Autodesk Inventor part; units mm, degrees
note: some values were not read from the file. Chosen so that the rebuilt part matches the saved one: direction of "Hole2".
(part 18 of 20)
  ellipse E641 centre (8.105457, -1.905648) end of major axis (8.046544, -1.401076) minor radius 0.000049 (8.046544, -1.401076) -> (8.078209, -1.672645) ccw
  line L861 (7.588206, -0.94314) -> (7.98763, -0.896503)
  line L862 (8.837388, -8.177544) -> (8.078209, -1.672645)
  line L863 (8.05096, -1.439642) -> (8.81014, -7.944541)
  line L864 (8.981303, -0.780694) -> (7.987731, -0.896542)
  line L865 (8.046645, -1.401115) -> (7.987731, -0.896542)
  line L866 (8.046645, -1.401115) -> (9.040217, -1.285266)
  line L867 (9.040217, -1.285266) -> (8.981303, -0.780694)
  line L868 (8.981373, -0.780721) -> (8.981303, -0.780694)
  line L869 (7.987731, -0.896542) -> (7.98763, -0.896503)
  line L870 (8.046544, -1.401076) -> (8.046645, -1.401115)
  line L871 (-7.593552, -4.618887) -> (-7.774689, -6.528342)
  line L872 (-7.593589, -4.618889) -> (-7.662654, -5.34695)
  ellipse E642 centre (-7.593625, -4.618891) end of major axis (-7.6416, -5.124621) minor radius 0.000036 (-7.593588, -4.618887) -> (-7.57144, -4.385367) ccw
  ellipse E643 centre (-7.593625, -4.618891) end of major axis (-7.689575, -5.63035) minor radius 0.000072 (-7.593552, -4.618882) -> (-7.549255, -4.151843) ccw
  ellipse E644 centre (-6.975368, 1.901046) end of major axis (-6.879418, 2.912506) minor radius 0.000072 (-6.930999, 2.36809) -> (-6.879418, 2.912506) ccw
  ellipse E645 centre (-6.975368, 1.901046) end of major axis (-6.927393, 2.406776) minor radius 0.000036 (-6.953183, 2.134568) -> (-6.927393, 2.406776) ccw
  line L873 (-6.879418, 2.912506) -> (-4.599252, 2.696203)
  line L874 (-7.57144, -4.385369) -> (-6.953183, 2.134568)
  line L875 (-7.549256, -4.151847) -> (-6.930999, 2.36809)
  line L876 (-6.87949, 2.912501) -> (-7.875247, 3.006926)
  line L877 (-7.923221, 2.501197) -> (-7.875247, 3.006926)
  line L878 (-7.923221, 2.501197) -> (-6.927464, 2.406772)
  line L879 (-6.87949, 2.912501) -> (-6.927464, 2.406772)
  line L880 (-7.875247, 3.006926) -> (-7.875359, 3.006919)
  line L881 (-6.927464, 2.406772) -> (-6.927393, 2.406776)
  line L882 (-6.879418, 2.912506) -> (-6.87949, 2.912501)
  line L883 (-3.994803, -3.77755) -> (-3.994871, -4.67207)
  line L884 (4.005197, -3.778158) -> (4.005129, -4.672679)
  line L885 (-3.994803, -3.77755) -> (-3.994768, -3.321333)
  line L886 (4.005197, -3.778158) -> (4.005231, -3.321941)
  line L887 (4.005703, 2.876499) -> (4.005738, 3.340448)
  line L888 (-3.994262, 3.341056) -> (-3.994297, 2.877107)
  line L889 (-3.994262, 3.341056) -> (4.005738, 3.340448)
  line L890 (-3.994768, -3.321333) -> (-3.994297, 2.877107)
  line L891 (4.005703, 2.876499) -> (4.005231, -3.321941)
  line L892 (5.005708, 2.94345) -> (4.005731, 3.241593)
  line L893 (4.005692, 2.735858) -> (4.482473, 2.593706)
  line L894 (5.005692, 2.732918) -> (5.005708, 2.94345)
  line L895 (-3.994269, 3.242201) -> (-4.994292, 2.94421)
  line L896 (-4.994308, 2.733679) -> (-4.994292, 2.94421)
  line L897 (-4.47111, 2.594387) -> (-3.994308, 2.736466)
  line L898 (7.672809, -5.348116) -> (7.603854, -4.620045)
  line L899 (7.603818, -4.620042) -> (7.784664, -6.529525)
  ellipse E646 centre (7.603891, -4.620047) end of major axis (7.555992, -4.11431) minor radius 0.000036 (7.581741, -4.386522) -> (7.603854, -4.620045) ccw
  ellipse E647 centre (7.603891, -4.620047) end of major axis (7.699687, -5.631521) minor radius 0.000072 (7.559592, -4.152992) -> (7.603817, -4.620038) ccw
  ellipse E648 centre (6.986625, 1.899985) end of major axis (6.890829, 2.911458) minor radius 0.000072 (6.890829, 2.911458) -> (6.942327, 2.367035) ccw
  ellipse E649 centre (6.986625, 1.899985) end of major axis (6.938727, 2.405721) minor radius 0.000036 (6.938727, 2.405721) -> (6.964476, 2.13351) ccw
  line L900 (4.610631, 2.695502) -> (6.890829, 2.911458)
  line L901 (7.581741, -4.386522) -> (6.964476, 2.13351)
  line L902 (6.942327, 2.367035) -> (7.559592, -4.152996)
  line L903 (7.886672, 3.005727) -> (6.890901, 2.911454)
  line L904 (6.938799, 2.405717) -> (6.890901, 2.911454)
  line L905 (6.938799, 2.405717) -> (7.93457, 2.499991)
  line L906 (7.93457, 2.499991) -> (7.886672, 3.005727)
  line L907 (7.886784, 3.00572) -> (7.886672, 3.005727)
  line L908 (6.890901, 2.911454) -> (6.890829, 2.911458)
  line L909 (6.938727, 2.405721) -> (6.938799, 2.405717)
  line L910 (-7.776794, -8.27734) -> (-7.755978, -8.078526)
  line L911 (-7.75575, -8.07845) -> (-7.776577, -8.277363)
  line L912 (-7.755978, -8.078526) -> (-7.75575, -8.07845)
  line L913 (-8.025217, -8.25133) -> (-8.025445, -8.251406)
  line L914 (-7.776577, -8.277363) -> (-8.025217, -8.25133)
  line L915 (-6.782013, -8.381497) -> (-6.761187, -8.182584)
  line L916 (-6.533372, -8.40753) -> (-6.782013, -8.381497)
  line L917 (-6.731454, -10.297276) -> (-6.979877, -10.271266)
  line L918 (-6.731226, -10.2972) -> (-6.731454, -10.297276)
  line L919 (-7.000693, -10.47008) -> (-6.979867, -10.271167)
  line L920 (-6.979867, -10.271167) -> (-6.731226, -10.2972)
  line L921 (-7.000922, -10.470155) -> (-7.000693, -10.47008)
  line L922 (-7.000922, -10.470155) -> (-7.265073, -10.442498)
  line L923 (-8.208069, -9.995621) -> (-8.025445, -8.251406)
  line L924 (-7.75575, -8.07845) -> (-6.761187, -8.182584)
  line L925 (-6.533372, -8.40753) -> (-6.731226, -10.2972)
  line L926 (-8.223071, -10.141) -> (-8.025217, -8.25133)
  line L927 (-7.000693, -10.47008) -> (-7.995257, -10.365946)
  line L928 (-8.223071, -10.141) -> (-7.97443, -10.167033)
  line L929 (-7.97443, -10.167033) -> (-7.995257, -10.365946)
  line L930 (-6.80284, -8.580409) -> (-6.95904, -10.072254)
  line L931 (-6.95904, -10.072254) -> (-7.953603, -9.968121)
  line L932 (-7.953603, -9.968121) -> (-7.797403, -8.476276)
  line L933 (-7.797403, -8.476276) -> (-6.80284, -8.580409)
  line L934 (-7.11621, -9.878579) -> (-6.996733, -8.73747)
  line L935 (-6.95904, -10.072254) -> (-7.11621, -9.878579)
  line L936 (-6.80284, -8.580409) -> (-6.996733, -8.73747)
  line L937 (-6.996733, -8.73747) -> (-7.640559, -8.67006)
  line L938 (-7.797403, -8.476276) -> (-7.640559, -8.67006)
  line L939 (-7.640559, -8.67006) -> (-7.760036, -9.811168)
  line L940 (-7.953603, -9.968121) -> (-7.760036, -9.811168)
  line L941 (-7.760036, -9.811168) -> (-7.11621, -9.878579)
  circle A21 centre (-7.35107, -9.013818) radius 0.1
  line L942 (-7.517123, -9.159232) -> (-7.483402, -8.83717)
  line L943 (-7.483435, -8.837181) -> (-7.483402, -8.83717)
  line L944 (-7.517156, -9.159243) -> (-7.483435, -8.837181)
  line L945 (-7.517156, -9.159243) -> (-7.517123, -9.159232)
  line L946 (-7.483402, -8.83717) -> (-7.185033, -8.86841)
  line L947 (-7.185033, -8.86841) -> (-7.218754, -9.190472)
  line L948 (-7.218787, -9.190483) -> (-7.218754, -9.190472)
  line L949 (-7.218754, -9.190472) -> (-7.517123, -9.159232)
  line L950 (-7.218787, -9.190483) -> (-7.517156, -9.159243)
  line L951 (-6.390906, -18.904533) -> (-6.589819, -18.883707)
  line L952 (-6.390678, -18.904457) -> (-6.390906, -18.904533)
  line L953 (-6.589591, -18.883631) -> (-6.390678, -18.904457)
  line L954 (-6.589819, -18.883707) -> (-6.589591, -18.883631)
  line L955 (-6.416939, -19.153174) -> (-6.390906, -18.904533)
  line L956 (-6.416711, -19.153098) -> (-6.416939, -19.153174)
  line L957 (-6.390678, -18.904457) -> (-6.416711, -19.153098)
  line L958 (-6.286762, -17.909871) -> (-6.260739, -17.661329)
  line L959 (-6.485457, -17.889067) -> (-6.485685, -17.889143)
  line L960 (-6.286544, -17.909894) -> (-6.485457, -17.889067)
  line L961 (-6.260511, -17.661253) -> (-6.286544, -17.909894)
  line L962 (-6.260739, -17.661329) -> (-6.260511, -17.661253)
  line L963 (-6.589819, -18.883707) -> (-6.485685, -17.889143)
  line L964 (-4.527269, -19.351028) -> (-6.416939, -19.153174)
  line L965 (-6.589591, -18.883631) -> (-6.485457, -17.889067)
  line L966 (-6.260511, -17.661253) -> (-4.370841, -17.859107)
  line L967 (-4.527041, -19.350952) -> (-6.416711, -19.153098)
  line L968 (-4.197961, -18.128574) -> (-4.302095, -19.123138)
  line L969 (-4.302323, -19.123214) -> (-4.501018, -19.10241)
  line L970 (-4.527041, -19.350952) -> (-4.501008, -19.102311)
  line L971 (-4.501008, -19.102311) -> (-4.302095, -19.123138)
  line L972 (-4.302095, -19.123138) -> (-4.302323, -19.123214)
  line L973 (-4.527269, -19.351028) -> (-4.527041, -19.350952)
  line L974 (-4.197961, -18.128574) -> (-4.396874, -18.107748)
  line L975 (-4.396874, -18.107748) -> (-4.370841, -17.859107)
  line L976 (-6.087632, -17.930721) -> (-4.595787, -18.086921)
  line L977 (-4.595787, -18.086921) -> (-4.69992, -19.081484)
  line L978 (-4.69992, -19.081484) -> (-6.191765, -18.925284)
  line L979 (-6.191765, -18.925284) -> (-6.087632, -17.930721)
  line L980 (-4.78968, -18.243982) -> (-5.930788, -18.124505)
  line L981 (-4.595787, -18.086921) -> (-4.78968, -18.243982)
  line L982 (-6.087632, -17.930721) -> (-5.930788, -18.124505)
  line L983 (-5.930788, -18.124505) -> (-5.998198, -18.768332)
  line L984 (-6.191765, -18.925284) -> (-5.998198, -18.768332)
  line L985 (-5.998198, -18.768332) -> (-4.85709, -18.887809)
  line L986 (-4.69992, -19.081484) -> (-4.85709, -18.887809)
  line L987 (-4.85709, -18.887809) -> (-4.78968, -18.243982)
  circle A22 centre (-5.654386, -18.47887) radius 0.1
  line L988 (-5.508983, -18.644917) -> (-5.831045, -18.611196)
  line L989 (-5.831077, -18.611207) -> (-5.831045, -18.611196)
  line L990 (-5.509015, -18.644928) -> (-5.831077, -18.611207)
  line L991 (-5.509015, -18.644928) -> (-5.508983, -18.644917)
  line L992 (-5.831045, -18.611196) -> (-5.799805, -18.312827)
  line L993 (-5.799837, -18.312838) -> (-5.799805, -18.312827)
  line L994 (-5.831077, -18.611207) -> (-5.799837, -18.312838)
  line L995 (-5.799805, -18.312827) -> (-5.477743, -18.346548)
  line L996 (-5.477743, -18.346548) -> (-5.508983, -18.644917)
  line L997 (-3.430044, -6.945819) -> (-3.430059, -7.144732)
  line L998 (-3.430059, -7.144732) -> (-3.680059, -7.144713)
  line L999 (-2.430059, -7.144809) -> (-2.430044, -6.945895)
  line L1000 (-2.180059, -7.144828) -> (-2.430059, -7.144809)
  line L1001 (-3.430044, -6.945819) -> (-2.430044, -6.945895)
  line L1002 (-2.180059, -7.144828) -> (-2.180193, -8.902773)
  line L1003 (-3.680193, -8.902659) -> (-3.680059, -7.144713)
  line L1004 (-2.430074, -7.343723) -> (-2.430178, -8.704102)
  line L1005 (-3.430178, -8.704026) -> (-3.430074, -7.343646)
  line L1006 (-3.430074, -7.343646) -> (-2.430074, -7.343723)
  line L1007 (-2.430074, -7.343723) -> (-2.590055, -7.597215)
  line L1008 (-3.430074, -7.343646) -> (-3.270133, -7.597163)
  ellipse E650 centre (-2.930117, -7.907177) end of major axis (-2.830117, -7.907184) minor radius 0.099457
  ellipse E651 centre (-2.930118, -7.91238) end of major axis (-2.830118, -7.912388) minor radius 0.099457 (-3.030118, -7.912373) -> (-2.830118, -7.912388) ccw
  line L1009 (-3.030118, -7.912373) -> (-3.030117, -7.907169)
  line L1010 (-2.830118, -7.912388) -> (-2.830117, -7.907184)
  line L1011 (-3.08013, -8.073401) -> (-3.080105, -7.751337)
  line L1012 (-3.080131, -8.083948) -> (-3.08013, -8.073401)
  line L1013 (-3.080105, -7.751337) -> (-2.780105, -7.751359)
  line L1014 (-2.780105, -7.751359) -> (-2.78013, -8.073424)
  line L1015 (-2.780131, -8.083971) -> (-2.78013, -8.073424)
  line L1016 (-2.78013, -8.073424) -> (-3.08013, -8.073401)
  line L1017 (-1.145848, -17.513296) -> (-0.945848, -17.513311)
  line L1018 (-1.145854, -17.595223) -> (-1.145848, -17.513296)
  line L1019 (-0.945867, -17.761954) -> (-0.945873, -17.843571)
  line L1020 (-0.945848, -17.513311) -> (-0.945867, -17.761954)
  line L1021 (-0.945772, -16.518742) -> (-1.145772, -16.518726)
  line L1022 (-0.945753, -16.270099) -> (-0.945772, -16.518742)
  line L1023 (-1.145848, -17.513296) -> (-1.145772, -16.518726)
  line L1024 (-0.945753, -16.270099) -> (0.954247, -16.270244)
  line L1025 (0.954133, -17.762098) -> (-0.945867, -17.761954)
  line L1026 (1.154228, -16.518901) -> (1.154152, -17.513471)
  line L1027 (0.954133, -17.762098) -> (0.954152, -17.513456)
  line L1028 (0.954152, -17.513456) -> (1.154152, -17.513471)
  line L1029 (1.154152, -17.513471) -> (1.154146, -17.595398)
  line L1030 (0.954127, -17.843715) -> (0.954133, -17.762098)
  line L1031 (1.154228, -16.518901) -> (0.954228, -16.518886)
  line L1032 (0.954228, -16.518886) -> (0.954247, -16.270244)
  line L1033 (-0.745772, -16.518757) -> (0.754228, -16.518871)
  line L1034 (0.754228, -16.518871) -> (0.754152, -17.513441)
  line L1035 (0.754152, -17.513441) -> (-0.745848, -17.513327)
  line L1036 (-0.745848, -17.513327) -> (-0.745772, -16.518757)
  line L1037 (0.754228, -16.518871) -> (0.613598, -16.741703)
  line L1038 (-0.745772, -16.518757) -> (-0.605176, -16.74161)
  line L1039 (-0.745848, -17.513327) -> (-0.606744, -17.457092)
  line L1040 (0.754152, -17.513441) -> (0.615057, -17.457185)
  ellipse E652 centre (-0.257727, -17.094133) end of major axis (-0.157727, -17.09414) minor radius 0.099457
  line L1041 (-0.357728, -17.098618) -> (-0.357727, -17.094125)
  line L1042 (-0.157728, -17.098634) -> (-0.157727, -17.09414)
  line L1043 (4.509081, -19.103095) -> (4.310383, -19.123869)
  line L1044 (4.310154, -19.123793) -> (4.50907, -19.102996)
  line L1045 (4.310383, -19.123869) -> (4.310154, -19.123793)
  line L1046 (4.535066, -19.351641) -> (4.535294, -19.351717)
  line L1047 (4.50907, -19.102996) -> (4.535066, -19.351641)
  line L1048 (4.405088, -18.108417) -> (4.206172, -18.129214)
  line L1049 (4.379093, -17.859772) -> (4.405088, -18.108417)
  line L1050 (6.269021, -17.662282) -> (6.295006, -17.910828)
  line L1051 (6.268793, -17.662206) -> (6.269021, -17.662282)
  line L1052 (6.493704, -17.890055) -> (6.294789, -17.910851)
  line L1053 (6.294789, -17.910851) -> (6.268793, -17.662206)
  line L1054 (6.493932, -17.89013) -> (6.493704, -17.890055)
  line L1055 (6.493932, -17.89013) -> (6.597915, -18.88471)
  line L1056 (6.424994, -19.154151) -> (4.535294, -19.351717)
  line L1057 (4.310154, -19.123793) -> (4.206172, -18.129214)
  line L1058 (4.379093, -17.859772) -> (6.268793, -17.662206)
  line L1059 (6.424766, -19.154075) -> (4.535066, -19.351641)
  line L1060 (6.493704, -17.890055) -> (6.597687, -18.884634)
  line L1061 (6.597915, -18.88471) -> (6.398999, -18.905506)
  line L1062 (6.398999, -18.905506) -> (6.424994, -19.154151)
  line L1063 (6.424766, -19.154075) -> (6.398771, -18.90543)
  line L1064 (6.398771, -18.90543) -> (6.597687, -18.884634)
  line L1065 (6.597687, -18.884634) -> (6.597915, -18.88471)
  line L1066 (6.398771, -18.90543) -> (6.398999, -18.905506)
  line L1067 (6.424994, -19.154151) -> (6.424766, -19.154075)
  line L1068 (4.604004, -18.087621) -> (6.095873, -17.931647)
  line L1069 (6.095873, -17.931647) -> (6.199855, -18.926227)
  line L1070 (6.199855, -18.926227) -> (4.707986, -19.0822)
  line L1071 (4.707986, -19.0822) -> (4.604004, -18.087621)
  line L1072 (5.938999, -18.125408) -> (4.797873, -18.244711)
  line L1073 (6.095873, -17.931647) -> (5.938999, -18.125408)
  line L1074 (4.604004, -18.087621) -> (4.797873, -18.244711)
  line L1075 (4.797873, -18.244711) -> (4.865185, -18.888548)
  line L1076 (4.707986, -19.0822) -> (4.865185, -18.888548)
  line L1077 (4.865185, -18.888548) -> (6.006312, -18.769245)
  line L1078 (6.199855, -18.926227) -> (6.006312, -18.769245)
  line L1079 (6.006312, -18.769245) -> (5.938999, -18.125408)
  circle A23 centre (5.14156, -18.534198) radius 0.1
  line L1080 (5.318199, -18.666552) -> (4.996132, -18.700224)
  line L1081 (4.996164, -18.700235) -> (4.996132, -18.700224)
  line L1082 (5.318232, -18.666563) -> (4.996164, -18.700235)
  line L1083 (5.318232, -18.666563) -> (5.318199, -18.666552)
  line L1084 (4.996132, -18.700224) -> (4.964937, -18.40185)
  line L1085 (4.964937, -18.40185) -> (5.287004, -18.368178)
  line L1086 (5.287037, -18.368189) -> (5.287004, -18.368178)
  line L1087 (5.287004, -18.368178) -> (5.318199, -18.666552)
  line L1088 (5.287037, -18.368189) -> (5.318232, -18.666563)
  line L1089 (-1.146141, -21.369416) -> (-0.946141, -21.369432)
  line L1090 (-0.946141, -21.369432) -> (-0.94616, -21.619432)
  line L1091 (-0.946065, -20.369432) -> (-1.146065, -20.369416)
  line L1092 (-0.946054, -20.223706) -> (-0.946065, -20.369432)
  line L1093 (-1.146141, -21.369416) -> (-1.146065, -20.369416)
  line L1094 (0.95384, -21.619576) -> (-0.94616, -21.619432)
  line L1095 (1.153935, -20.369591) -> (1.153859, -21.369591)
  line L1096 (0.95384, -21.619576) -> (0.953859, -21.369576)
  line L1097 (0.953859, -21.369576) -> (1.153859, -21.369591)
  line L1098 (1.153935, -20.369591) -> (0.953935, -20.369576)
  line L1099 (0.953935, -20.369576) -> (0.953946, -20.22385)
  line L1100 (-0.746065, -20.369447) -> (0.753935, -20.369561)
  line L1101 (0.753935, -20.369561) -> (0.753859, -21.369561)
  line L1102 (0.753859, -21.369561) -> (-0.746141, -21.369447)
  line L1103 (-0.746141, -21.369447) -> (-0.746065, -20.369447)
  line L1104 (0.577595, -20.545874) -> (-0.569751, -20.545787)
  line L1105 (0.753935, -20.369561) -> (0.577595, -20.545874)
  line L1106 (-0.746065, -20.369447) -> (-0.569751, -20.545787)
  line L1107 (-0.569751, -20.545787) -> (-0.569801, -21.193133)
  line L1108 (-0.746141, -21.369447) -> (-0.569801, -21.193133)
  line L1109 (-0.569801, -21.193133) -> (0.577545, -21.193221)
  line L1110 (0.753859, -21.369561) -> (0.577545, -21.193221)
  line L1111 (0.577545, -21.193221) -> (0.577595, -20.545874)
  circle A24 centre (-0.258014, -20.869484) radius 0.1
  line L1112 (-0.096114, -21.019496) -> (-0.419937, -21.019472)
  line L1113 (-0.419937, -21.019472) -> (-0.419914, -20.719472)
  line L1114 (-0.419914, -20.719472) -> (-0.096092, -20.719496)
  line L1115 (-0.096092, -20.719496) -> (-0.096114, -21.019496)
  line L1116 (-1.146233, -22.580088) -> (-0.946233, -22.580104)
  line L1117 (-0.946233, -22.580104) -> (-0.946252, -22.828417)
  line L1118 (-1.146233, -22.580088) -> (-1.146198, -22.119416)
  line L1119 (0.953748, -22.828561) -> (-0.946252, -22.828417)
  line L1120 (1.153802, -22.119591) -> (1.153767, -22.580263)
  line L1121 (0.953748, -22.828561) -> (0.953767, -22.580248)
  line L1122 (0.953767, -22.580248) -> (1.153767, -22.580263)
  line L1123 (0.753802, -22.119561) -> (0.753767, -22.580233)
  line L1124 (0.753767, -22.580233) -> (-0.746233, -22.580119)
  line L1125 (-0.746233, -22.580119) -> (-0.746198, -22.119447)
  line L1126 (-0.569871, -22.11946) -> (-0.569884, -22.289016)
  line L1127 (-0.746233, -22.580119) -> (-0.569884, -22.289016)
  line L1128 (-0.569884, -22.289016) -> (0.577462, -22.289103)
  line L1129 (0.753767, -22.580233) -> (0.577462, -22.289103)
  line L1130 (0.577462, -22.289103) -> (0.577475, -22.119548)
  line L1131 (-0.0962, -22.139747) -> (-0.420022, -22.139722)
  line L1132 (-0.420022, -22.139722) -> (-0.420021, -22.119472)
  line L1133 (-0.096198, -22.119496) -> (-0.0962, -22.139747)
  line L1134 (-8.467791, -9.965256) -> (-8.491015, -10.163903)
  line L1135 (-8.467932, -9.96531) -> (-8.467791, -9.965256)
  line L1136 (-8.739324, -10.134872) -> (-8.739466, -10.134927)
  line L1137 (-8.491015, -10.163903) -> (-8.739324, -10.134872)
  line L1138 (-8.707345, -12.252986) -> (-8.735015, -12.249751)
  line L1139 (-8.960099, -12.022073) -> (-8.739466, -10.134927)
  line L1140 (-8.467791, -9.965256) -> (-8.207852, -9.995646)
  line L1141 (-7.265061, -10.4424) -> (-7.470105, -12.196203)
  line L1142 (-8.959957, -12.022019) -> (-8.739324, -10.134872)
  line L1143 (-7.741638, -12.365819) -> (-8.734873, -12.249696)
  line L1144 (-8.735015, -12.249751) -> (-8.723713, -12.15308)
  line L1145 (-8.739665, -12.047845) -> (-8.960099, -12.022073)
  line L1146 (-8.959957, -12.022019) -> (-8.711649, -12.051049)
  line L1147 (-8.711649, -12.051049) -> (-8.734873, -12.249696)
  line L1148 (-8.734873, -12.249696) -> (-8.735015, -12.249751)
  line L1149 (-8.711649, -12.051049) -> (-8.71179, -12.051104)
  line L1150 (-8.960099, -12.022073) -> (-8.959957, -12.022019)
  line L1151 (-7.470105, -12.196203) -> (-7.470246, -12.196257)
  line L1152 (-7.741638, -12.365819) -> (-7.718414, -12.167172)
  line L1153 (-7.718414, -12.167172) -> (-7.470105, -12.196203)
  line L1154 (-7.74178, -12.365873) -> (-7.741638, -12.365819)
  line L1155 (-7.521005, -10.478673) -> (-7.695189, -11.968525)
  line L1156 (-7.695189, -11.968525) -> (-8.688424, -11.852402)
  line L1157 (-8.688424, -11.852402) -> (-8.51424, -10.36255)
  line L1158 (-8.51424, -10.36255) -> (-7.521005, -10.478673)
  line L1159 (-7.849949, -11.772954) -> (-7.716716, -10.63337)
  line L1160 (-7.695189, -11.968525) -> (-7.849949, -11.772954)
  line L1161 (-7.521005, -10.478673) -> (-7.716716, -10.63337)
  line L1162 (-7.716716, -10.63337) -> (-8.359683, -10.558199)
  line L1163 (-8.51424, -10.36255) -> (-8.359683, -10.558199)
  line L1164 (-8.359683, -10.558199) -> (-8.492916, -11.697783)
  line L1165 (-8.688424, -11.852402) -> (-8.492916, -11.697783)
  line L1166 (-8.492916, -11.697783) -> (-7.849949, -11.772954)
  circle A25 centre (-8.074377, -10.905427) radius 0.1
  line L1167 (-8.242168, -11.048827) -> (-8.204565, -10.727195)
  line L1168 (-8.204585, -10.727202) -> (-8.204565, -10.727195)
  line L1169 (-8.242189, -11.048835) -> (-8.204585, -10.727202)
  line L1170 (-8.242189, -11.048835) -> (-8.242168, -11.048827)
  line L1171 (-8.204565, -10.727195) -> (-7.906595, -10.762032)
  line L1172 (-7.906595, -10.762032) -> (-7.944198, -11.083664)
  line L1173 (-7.944218, -11.083671) -> (-7.944198, -11.083664)
  line L1174 (-7.944198, -11.083664) -> (-8.242168, -11.048827)
  line L1175 (-7.944218, -11.083671) -> (-8.242189, -11.048835)
  line L1176 (-7.233548, -20.806996) -> (-7.432195, -20.783772)
  line L1177 (-7.233407, -20.806942) -> (-7.233548, -20.806996)
  line L1178 (-7.432054, -20.783717) -> (-7.233407, -20.806942)
  line L1179 (-7.432195, -20.783772) -> (-7.432054, -20.783717)
  line L1180 (-7.262579, -21.055305) -> (-7.233548, -20.806996)
  line L1181 (-7.262437, -21.05525) -> (-7.262579, -21.055305)
  line L1182 (-7.233407, -20.806942) -> (-7.262437, -21.05525)
  line L1183 (-7.117417, -19.813691) -> (-7.090722, -19.585361)
  line L1184 (-7.315931, -19.790482) -> (-7.316072, -19.790537)
  line L1185 (-7.117284, -19.813707) -> (-7.315931, -19.790482)
  line L1186 (-7.088253, -19.565398) -> (-7.117284, -19.813707)
  line L1187 (-7.088395, -19.565452) -> (-7.088253, -19.565398)
  line L1188 (-7.432195, -20.783772) -> (-7.316072, -19.790537)
  line L1189 (-5.375433, -21.275938) -> (-7.262579, -21.055305)
  line L1190 (-7.432054, -20.783717) -> (-7.315931, -19.790482)
  line L1191 (-7.088253, -19.565398) -> (-5.201107, -19.786031)
  line L1192 (-5.375291, -21.275884) -> (-7.262437, -21.05525)
  line L1193 (-5.031491, -20.057565) -> (-5.147613, -21.050799)
  line L1194 (-5.147755, -21.050854) -> (-5.346269, -21.027645)
  line L1195 (-5.375291, -21.275884) -> (-5.34626, -21.027575)
  line L1196 (-5.34626, -21.027575) -> (-5.147613, -21.050799)
  line L1197 (-5.147613, -21.050799) -> (-5.147755, -21.050854)
  line L1198 (-5.375433, -21.275938) -> (-5.375291, -21.275884)
  line L1199 (-5.031491, -20.057565) -> (-5.230138, -20.03434)
  line L1200 (-5.230138, -20.03434) -> (-5.201107, -19.786031)
  line L1201 (-6.918637, -19.836931) -> (-5.428785, -20.011115)
  line L1202 (-5.428785, -20.011115) -> (-5.544907, -21.00435)
  line L1203 (-5.544907, -21.00435) -> (-7.03476, -20.830166)
  line L1204 (-7.03476, -20.830166) -> (-6.918637, -19.836931)
  line L1205 (-5.624495, -20.165813) -> (-6.76408, -20.03258)
  line L1206 (-5.428785, -20.011115) -> (-5.624495, -20.165813)
  line L1207 (-6.918637, -19.836931) -> (-6.76408, -20.03258)
  line L1208 (-6.76408, -20.03258) -> (-6.839251, -20.675547)
  line L1209 (-7.03476, -20.830166) -> (-6.839251, -20.675547)
  line L1210 (-6.839251, -20.675547) -> (-5.699667, -20.80878)
  line L1211 (-5.544907, -21.00435) -> (-5.699667, -20.80878)
  line L1212 (-5.699667, -20.80878) -> (-5.624495, -20.165813)
  circle A26 centre (-6.491988, -20.390256) radius 0.1
  line L1213 (-6.348595, -20.558045) -> (-6.670227, -20.520442)
  line L1214 (-6.670247, -20.520449) -> (-6.670227, -20.520442)
  line L1215 (-6.348615, -20.558053) -> (-6.670247, -20.520449)
  line L1216 (-6.348615, -20.558053) -> (-6.348595, -20.558045)
  line L1217 (-6.670227, -20.520442) -> (-6.63539, -20.222471)
  line L1218 (-6.63541, -20.222479) -> (-6.63539, -20.222471)
  line L1219 (-6.670247, -20.520449) -> (-6.63541, -20.222479)
  line L1220 (-6.63539, -20.222471) -> (-6.313758, -20.260074)
  line L1221 (-6.313758, -20.260074) -> (-6.348595, -20.558045)
  line L1222 (-3.430178, -8.704026) -> (-3.430193, -8.902678)
  line L1223 (-3.430193, -8.902678) -> (-3.680193, -8.902659)
  line L1224 (-2.430193, -8.902754) -> (-2.430178, -8.704102)
  line L1225 (-2.180193, -8.902773) -> (-2.430193, -8.902754)
  line L1226 (-2.180349, -10.95225) -> (-2.430349, -10.952231)
  line L1227 (-2.180336, -10.789965) -> (-2.180349, -10.95225)
  line L1228 (-2.430352, -10.988597) -> (-2.430336, -10.789946)
  line L1229 (-2.430336, -10.789946) -> (-2.180336, -10.789965)
  line L1230 (-2.430364, -11.150883) -> (-2.430352, -10.988597)
  line L1231 (-2.430364, -11.150883) -> (-3.430364, -11.150807)
  line L1232 (-3.430178, -8.704026) -> (-2.430178, -8.704102)
  line L1233 (-2.180193, -8.902773) -> (-2.180336, -10.789965)
  line L1234 (-3.680336, -10.789851) -> (-3.680193, -8.902659)
  line L1235 (-2.430352, -10.988597) -> (-3.430352, -10.988521)
  line L1236 (-3.430349, -10.952155) -> (-3.680349, -10.952136)
  line L1237 (-3.680336, -10.789851) -> (-3.430336, -10.78987)
  line L1238 (-3.430336, -10.78987) -> (-3.430352, -10.988521)
  line L1239 (-3.430352, -10.988521) -> (-3.430364, -11.150807)
  line L1240 (-3.680349, -10.952136) -> (-3.680336, -10.789851)
  line L1241 (-2.430208, -9.101406) -> (-2.430321, -10.591294)
  line L1242 (-2.430321, -10.591294) -> (-3.430321, -10.591218)
  line L1243 (-3.430321, -10.591218) -> (-3.430208, -9.10133)
  line L1244 (-3.430208, -9.10133) -> (-2.430208, -9.101406)
  line L1245 (-2.606644, -10.53206) -> (-2.606557, -9.392449)
  line L1246 (-2.430321, -10.591294) -> (-2.606644, -10.53206)
  line L1247 (-2.430208, -9.101406) -> (-2.606557, -9.392449)
  line L1248 (-2.606557, -9.392449) -> (-3.253903, -9.3924)
  line L1249 (-3.430208, -9.10133) -> (-3.253903, -9.3924)
  line L1250 (-3.253903, -9.3924) -> (-3.25399, -10.532011)
  line L1251 (-3.430321, -10.591218) -> (-3.25399, -10.532011)
  line L1252 (-3.25399, -10.532011) -> (-2.606644, -10.53206)
  ellipse E653 centre (-2.930252, -9.673105) end of major axis (-2.830252, -9.673112) minor radius 0.099326
  ellipse E654 centre (-2.930252, -9.678901) end of major axis (-2.830252, -9.678908) minor radius 0.099326 (-3.030252, -9.678893) -> (-2.830252, -9.678908) ccw
  line L1253 (-3.030252, -9.678893) -> (-3.030252, -9.673097)
  line L1254 (-2.830252, -9.678908) -> (-2.830252, -9.673112)
  line L1255 (-3.080264, -9.839709) -> (-3.08024, -9.518069)
  line L1256 (-3.080266, -9.862893) -> (-3.080264, -9.839709)
  line L1257 (-3.08024, -9.518069) -> (-2.78024, -9.518092)
  line L1258 (-2.78024, -9.518092) -> (-2.780264, -9.839732)
  line L1259 (-2.780266, -9.862916) -> (-2.780264, -9.839732)
  line L1260 (-2.780264, -9.839732) -> (-3.080264, -9.839709)
  line L1261 (-2.780266, -9.862916) -> (-3.080266, -9.862893)
  line L1262 (-0.945993, -19.419875) -> (-1.145993, -19.41986)
  line L1263 (-1.14598, -19.257574) -> (-0.94598, -19.257589)
  line L1264 (-1.145993, -19.41986) -> (-1.14598, -19.257574)
  line L1265 (-0.945999, -19.505904) -> (-0.946012, -19.66819)
  line L1266 (-0.94598, -19.257589) -> (-0.945999, -19.505904)
  line L1267 (-0.945905, -18.264331) -> (-1.145905, -18.264315)
  line L1268 (-0.945886, -18.016016) -> (-0.945905, -18.264331)
  line L1269 (1.154007, -19.420035) -> (0.954007, -19.420019)
  line L1270 (0.954001, -19.506049) -> (0.95402, -19.257734)
  line L1271 (0.95402, -19.257734) -> (1.15402, -19.257749)
  line L1272 (1.15402, -19.257749) -> (1.154007, -19.420035)
  line L1273 (0.953988, -19.668334) -> (0.954001, -19.506049)
  line L1274 (0.953988, -19.668334) -> (-0.946012, -19.66819)
  line L1275 (-1.14598, -19.257574) -> (-1.145905, -18.264315)
  line L1276 (-0.945886, -18.016016) -> (0.954114, -18.016161)
  line L1277 (0.954001, -19.506049) -> (-0.945999, -19.505904)
  line L1278 (1.154095, -18.26449) -> (1.15402, -19.257749)
  line L1279 (1.154095, -18.26449) -> (0.954095, -18.264475)
  line L1280 (0.954095, -18.264475) -> (0.954114, -18.016161)
  line L1281 (-0.745905, -18.264346) -> (0.754095, -18.26446)
  line L1282 (0.754095, -18.26446) -> (0.75402, -19.257719)
  line L1283 (0.75402, -19.257719) -> (-0.74598, -19.257605)
  line L1284 (-0.74598, -19.257605) -> (-0.745905, -18.264346)
  line L1285 (0.577746, -18.555503) -> (-0.5696, -18.555416)
  line L1286 (0.754095, -18.26446) -> (0.577746, -18.555503)
  line L1287 (-0.745905, -18.264346) -> (-0.5696, -18.555416)
  line L1288 (-0.5696, -18.555416) -> (-0.569649, -19.198398)
  line L1289 (-0.74598, -19.257605) -> (-0.569649, -19.198398)
  line L1290 (-0.569649, -19.198398) -> (0.577697, -19.198485)
  line L1291 (0.75402, -19.257719) -> (0.577697, -19.198485)
  line L1292 (0.577697, -19.198485) -> (0.577746, -18.555503)
  ellipse E655 centre (-0.257861, -18.847951) end of major axis (-0.157861, -18.847959) minor radius 0.099326
  ellipse E656 centre (-0.257861, -18.853747) end of major axis (-0.157861, -18.853755) minor radius 0.099326 (-0.357861, -18.853739) -> (-0.157861, -18.853755) ccw
  line L1293 (-0.357861, -18.853739) -> (-0.357861, -18.847943)
  line L1294 (-0.157861, -18.853755) -> (-0.157861, -18.847959)
  line L1295 (-0.095961, -19.002748) -> (-0.419784, -19.002723)
  line L1296 (-0.419786, -19.025907) -> (-0.419784, -19.002723)
  line L1297 (-0.095963, -19.025932) -> (-0.419786, -19.025907)
  line L1298 (-0.095963, -19.025932) -> (-0.095961, -19.002748)
  line L1299 (-0.419784, -19.002723) -> (-0.419761, -18.704746)
  line L1300 (-0.419761, -18.704746) -> (-0.095938, -18.70477)
  line L1301 (-0.095938, -18.70477) -> (-0.095961, -19.002748)
  line L1302 (5.354039, -21.028459) -> (5.155521, -21.051637)
  line L1303 (5.15538, -21.051583) -> (5.35403, -21.028389)
  line L1304 (5.155521, -21.051637) -> (5.15538, -21.051583)
  line L1305 (5.383023, -21.276702) -> (5.383165, -21.276756)
  line L1306 (5.35403, -21.028389) -> (5.383023, -21.276702)
  line L1307 (5.238059, -20.035136) -> (5.039408, -20.05833)
  line L1308 (5.209066, -19.786823) -> (5.238059, -20.035136)
  line L1309 (7.098712, -19.58644) -> (7.125372, -19.814774)
  line L1310 (7.096246, -19.566477) -> (7.096387, -19.566531)
  line L1311 (7.323889, -19.791595) -> (7.125238, -19.81479)
  line L1312 (7.125238, -19.81479) -> (7.096246, -19.566477)
  line L1313 (7.32403, -19.79165) -> (7.323889, -19.791595)
  line L1314 (7.32403, -19.79165) -> (7.440002, -20.784903)
  line L1315 (7.270345, -21.05641) -> (5.383165, -21.276756)
  line L1316 (5.15538, -21.051583) -> (5.039408, -20.05833)
  line L1317 (5.209066, -19.786823) -> (7.096246, -19.566477)
  line L1318 (7.270203, -21.056355) -> (5.383023, -21.276702)
  line L1319 (7.323889, -19.791595) -> (7.439861, -20.784848)
  line L1320 (7.440002, -20.784903) -> (7.241352, -20.808097)
  line L1321 (7.241352, -20.808097) -> (7.270345, -21.05641)
  line L1322 (7.270203, -21.056355) -> (7.24121, -20.808042)
  line L1323 (7.24121, -20.808042) -> (7.439861, -20.784848)
  line L1324 (7.439861, -20.784848) -> (7.440002, -20.784903)
  line L1325 (7.24121, -20.808042) -> (7.241352, -20.808097)
  line L1326 (7.270345, -21.05641) -> (7.270203, -21.056355)
  line L1327 (5.436709, -20.011942) -> (6.926588, -19.837984)
  line L1328 (6.926588, -19.837984) -> (7.04256, -20.831237)
  line L1329 (7.04256, -20.831237) -> (5.552681, -21.005194)
  line L1330 (5.552681, -21.005194) -> (5.436709, -20.011942)
  line L1331 (6.772001, -20.033609) -> (5.632396, -20.166669)
  line L1332 (6.926588, -19.837984) -> (6.772001, -20.033609)
  line L1333 (5.436709, -20.011942) -> (5.632396, -20.166669)
  line L1334 (5.632396, -20.166669) -> (5.70747, -20.809647)
  line L1335 (5.552681, -21.005194) -> (5.70747, -20.809647)
  line L1336 (5.70747, -20.809647) -> (6.847075, -20.676587)
  line L1337 (7.04256, -20.831237) -> (6.847075, -20.676587)
  line L1338 (6.847075, -20.676587) -> (6.772001, -20.033609)
  circle A27 centre (5.979566, -20.451993) radius 0.1
  line L1339 (6.157786, -20.582205) -> (5.836148, -20.61976)
  line L1340 (5.836168, -20.619767) -> (5.836148, -20.61976)
  line L1341 (6.157806, -20.582213) -> (5.836168, -20.619767)
  line L1342 (6.157806, -20.582213) -> (6.157786, -20.582205)
  line L1343 (5.836148, -20.61976) -> (5.801357, -20.321784)
  line L1344 (5.801357, -20.321784) -> (6.122994, -20.28423)
  line L1345 (6.123015, -20.284237) -> (6.122994, -20.28423)
  line L1346 (6.122994, -20.28423) -> (6.157786, -20.582205)
  line L1347 (6.123015, -20.284237) -> (6.157806, -20.582213)
  line L1348 (-7.191687, -6.365321) -> (-7.172801, -6.166231)
  line L1349 (-7.172701, -6.166225) -> (-7.191589, -6.365331)
  line L1350 (-7.172801, -6.166231) -> (-7.172701, -6.166225)
  line L1351 (-7.440471, -6.341721) -> (-7.440572, -6.341727)
  line L1352 (-7.191589, -6.365331) -> (-7.440471, -6.341721)
  line L1353 (-6.196058, -6.45977) -> (-6.17717, -6.260664)
  line L1354 (-5.947175, -6.483379) -> (-6.196058, -6.45977)
  line L1355 (-7.461453, -6.561848) -> (-7.440572, -6.341727)
  line L1356 (-7.172701, -6.166225) -> (-6.17717, -6.260664)
  line L1357 (-5.947175, -6.483379) -> (-6.126609, -8.374888)
  line L1358 (-7.606703, -8.094056) -> (-7.440471, -6.341721)
  line L1359 (-6.39438, -8.550384) -> (-6.546816, -8.535924)
  line L1360 (-6.126609, -8.374888) -> (-6.126709, -8.374894)
  line L1361 (-6.39438, -8.550384) -> (-6.375492, -8.351278)
  line L1362 (-6.375492, -8.351278) -> (-6.126609, -8.374888)
  line L1363 (-6.39448, -8.55039) -> (-6.39438, -8.550384)
  line L1364 (-6.214946, -6.658876) -> (-6.356604, -8.152172)
  line L1365 (-6.356604, -8.152172) -> (-7.352135, -8.057733)
  line L1366 (-7.352135, -8.057733) -> (-7.210476, -6.564437)
  line L1367 (-7.210476, -6.564437) -> (-6.214946, -6.658876)
  line L1368 (-6.515562, -7.959985) -> (-6.407208, -6.817767)
  line L1369 (-6.356604, -8.152172) -> (-6.515562, -7.959985)
  line L1370 (-6.214946, -6.658876) -> (-6.407208, -6.817767)
  line L1371 (-6.407208, -6.817767) -> (-7.051661, -6.756632)
  line L1372 (-7.210476, -6.564437) -> (-7.051661, -6.756632)
  line L1373 (-7.051661, -6.756632) -> (-7.160015, -7.89885)
  line L1374 (-7.352135, -8.057733) -> (-7.160015, -7.89885)
  line L1375 (-7.160015, -7.89885) -> (-6.515562, -7.959985)
  circle A28 centre (-6.758859, -7.097567) radius 0.1
  line L1376 (-6.923483, -7.244589) -> (-6.892902, -6.922213)
  line L1377 (-6.923498, -7.24459) -> (-6.892916, -6.922214)
  line L1378 (-6.892902, -6.922213) -> (-6.594243, -6.950545)
  line L1379 (-6.594243, -6.950545) -> (-6.624824, -7.272921)
  line L1380 (-6.624824, -7.272921) -> (-6.923483, -7.244589)
  line L1381 (-5.70222, -16.978419) -> (-5.70232, -16.978425)
  line L1382 (-5.901326, -16.959531) -> (-5.70222, -16.978419)
  line L1383 (-5.901427, -16.959537) -> (-5.901326, -16.959531)
  line L1384 (-5.72583, -17.227301) -> (-5.72593, -17.227307)
  line L1385 (-5.70222, -16.978419) -> (-5.72583, -17.227301)
  line L1386 (-5.806887, -15.964) -> (-5.806988, -15.964006)
  line L1387 (-5.607781, -15.982888) -> (-5.806887, -15.964)
  line L1388 (-5.584172, -15.734005) -> (-5.607781, -15.982888)
  line L1389 (-5.584272, -15.734011) -> (-5.584172, -15.734005)
  line L1390 (-5.901326, -16.959531) -> (-5.806887, -15.964)
  line L1391 (-5.584172, -15.734005) -> (-3.692663, -15.913439)
  line L1392 (-3.834322, -17.406735) -> (-5.72583, -17.227301)
  line L1393 (-3.517167, -16.181209) -> (-3.611606, -17.17674)
  line L1394 (-3.834322, -17.406735) -> (-3.810712, -17.157852)
  line L1395 (-3.810712, -17.157852) -> (-3.611606, -17.17674)
  line L1396 (-3.611606, -17.17674) -> (-3.611706, -17.176746)
  line L1397 (-3.834422, -17.406741) -> (-3.834322, -17.406735)
  line L1398 (-3.517167, -16.181209) -> (-3.716273, -16.162322)
  line L1399 (-3.716273, -16.162322) -> (-3.692663, -15.913439)
  line L1400 (-5.408675, -16.001776) -> (-3.915379, -16.143434)
  line L1401 (-3.915379, -16.143434) -> (-4.009818, -17.138965)
  line L1402 (-4.009818, -17.138965) -> (-5.503114, -16.997306)
  line L1403 (-5.503114, -16.997306) -> (-5.408675, -16.001776)
  line L1404 (-4.107642, -16.302325) -> (-5.24986, -16.193971)
  line L1405 (-3.915379, -16.143434) -> (-4.107642, -16.302325)
  line L1406 (-5.408675, -16.001776) -> (-5.24986, -16.193971)
  line L1407 (-5.24986, -16.193971) -> (-5.310995, -16.838424)
  line L1408 (-5.503114, -16.997306) -> (-5.310995, -16.838424)
  line L1409 (-5.310995, -16.838424) -> (-4.168776, -16.946778)
  line L1410 (-4.009818, -17.138965) -> (-4.168776, -16.946778)
  line L1411 (-4.168776, -16.946778) -> (-4.107642, -16.302325)
  circle A29 centre (-4.970041, -16.545639) radius 0.1
  line L1412 (-4.823023, -16.710259) -> (-5.145398, -16.679678)
  line L1413 (-5.145398, -16.679678) -> (-5.117067, -16.381019)
  line L1414 (-5.145413, -16.679679) -> (-5.117081, -16.38102)
  line L1415 (-5.117067, -16.381019) -> (-4.794691, -16.4116)
  line L1416 (-4.794691, -16.4116) -> (-4.823023, -16.710259)
  line L1417 (-3.429907, -5.13954) -> (-3.429922, -5.338648)
  line L1418 (-3.429922, -5.338648) -> (-3.679922, -5.338629)
  line L1419 (-2.429922, -5.338724) -> (-2.429907, -5.139616)
  line L1420 (-2.179922, -5.338743) -> (-2.429922, -5.338724)
  line L1421 (-3.429907, -5.13954) -> (-2.429907, -5.139616)
  line L1422 (-2.179922, -5.338743) -> (-2.180059, -7.144828)
  line L1423 (-3.680059, -7.144713) -> (-3.679922, -5.338629)
  line L1424 (-2.429937, -5.537833) -> (-2.430044, -6.945895)
  line L1425 (-3.430044, -6.945819) -> (-3.429937, -5.537757)
  line L1426 (-3.429937, -5.537757) -> (-2.429937, -5.537833)
  line L1427 (-2.606321, -6.288385) -> (-2.606285, -5.807685)
  line L1428 (-2.429937, -5.537833) -> (-2.606285, -5.807685)
  line L1429 (-2.606285, -5.807685) -> (-3.253631, -5.807636)
  line L1430 (-3.429937, -5.537757) -> (-3.253631, -5.807636)
  line L1431 (-3.253631, -5.807636) -> (-3.253667, -6.288336)
  ellipse E657 centre (-2.929979, -6.094451) end of major axis (-2.829979, -6.094458) minor radius 0.099554
  ellipse E658 centre (-2.92998, -6.099167) end of major axis (-2.82998, -6.099175) minor radius 0.099554 (-3.02998, -6.099159) -> (-2.82998, -6.099175) ccw
  line L1432 (-3.02998, -6.099159) -> (-3.029979, -6.094443)
  line L1433 (-2.82998, -6.099175) -> (-2.829979, -6.094458)
  line L1434 (-3.079992, -6.260345) -> (-3.079967, -5.937966)
  line L1435 (-3.079993, -6.27921) -> (-3.079992, -6.260345)
  line L1436 (-3.079967, -5.937966) -> (-2.779967, -5.937989)
  line L1437 (-2.779967, -5.937989) -> (-2.779992, -6.260368)
  line L1438 (-2.779993, -6.279233) -> (-2.779992, -6.260368)
  line L1439 (-2.779992, -6.260368) -> (-3.079992, -6.260345)
  line L1440 (-2.779993, -6.279233) -> (-3.079993, -6.27921)
  line L1441 (-1.145711, -15.717342) -> (-0.945711, -15.717357)
  line L1442 (-1.145713, -15.747824) -> (-1.145711, -15.717342)
  line L1443 (-0.94573, -15.966242) -> (-0.945732, -15.996212)
  line L1444 (-0.945711, -15.717357) -> (-0.94573, -15.966242)
  line L1445 (-0.945635, -14.721816) -> (-1.145635, -14.7218)
  line L1446 (-0.945617, -14.47293) -> (-0.945635, -14.721816)
  line L1447 (-1.145711, -15.717342) -> (-1.145635, -14.7218)
  line L1448 (-0.945617, -14.47293) -> (0.954383, -14.473075)
  line L1449 (0.95427, -15.966387) -> (-0.94573, -15.966242)
  line L1450 (1.154365, -14.721975) -> (1.154289, -15.717517)
  line L1451 (0.95427, -15.966387) -> (0.954289, -15.717501)
  line L1452 (0.954289, -15.717501) -> (1.154289, -15.717517)
  line L1453 (1.154289, -15.717517) -> (1.154286, -15.747999)
  line L1454 (0.954268, -15.996357) -> (0.95427, -15.966387)
  line L1455 (1.154365, -14.721975) -> (0.954365, -14.72196)
  line L1456 (0.954365, -14.72196) -> (0.954383, -14.473075)
  line L1457 (-0.745635, -14.721831) -> (0.754365, -14.721945)
  line L1458 (0.754365, -14.721945) -> (0.754289, -15.717486)
  line L1459 (0.754289, -15.717486) -> (-0.745711, -15.717372)
  line L1460 (-0.745711, -15.717372) -> (-0.745635, -14.721831)
  line L1461 (0.754365, -14.721945) -> (0.693778, -14.814656)
  line L1462 (-0.745635, -14.721831) -> (-0.685063, -14.814551)
  line L1463 (-0.745711, -15.717372) -> (-0.688508, -15.69103)
  line L1464 (0.754289, -15.717486) -> (0.69709, -15.691135)
  line L1465 (3.619961, -17.17729) -> (3.81907, -17.158433)
  line L1466 (3.620062, -17.177296) -> (3.619961, -17.17729)
  line L1467 (3.842642, -17.407319) -> (3.842743, -17.407325)
  line L1468 (3.81907, -17.158433) -> (3.842642, -17.407319)
  line L1469 (3.724783, -16.162888) -> (3.525674, -16.181745)
  line L1470 (3.701211, -15.914001) -> (3.724783, -16.162888)
  line L1471 (3.619961, -17.17729) -> (3.525674, -16.181745)
  line L1472 (3.701211, -15.914001) -> (5.592747, -15.734855)
  line L1473 (5.734178, -17.228173) -> (3.842642, -17.407319)
  line L1474 (5.815428, -15.964884) -> (5.909715, -16.960429)
  line L1475 (5.592747, -15.734855) -> (5.592847, -15.734861)
  line L1476 (5.815428, -15.964884) -> (5.616319, -15.983741)
  line L1477 (5.616319, -15.983741) -> (5.592747, -15.734855)
  line L1478 (5.815528, -15.96489) -> (5.815428, -15.964884)
  line L1479 (5.734178, -17.228173) -> (5.710606, -16.979286)
  line L1480 (5.710606, -16.979286) -> (5.909715, -16.960429)
  line L1481 (5.909715, -16.960429) -> (5.909815, -16.960435)
  line L1482 (5.710606, -16.979286) -> (5.710706, -16.979293)
  line L1483 (5.734278, -17.228179) -> (5.734178, -17.228173)
  line L1484 (3.923892, -16.14403) -> (5.41721, -16.002599)
  line L1485 (5.41721, -16.002599) -> (5.511497, -16.998144)
  line L1486 (5.511497, -16.998144) -> (4.018179, -17.139575)
  line L1487 (4.018179, -17.139575) -> (3.923892, -16.14403)
  line L1488 (5.258365, -16.19477) -> (4.11613, -16.302951)
  line L1489 (5.41721, -16.002599) -> (5.258365, -16.19477)
  line L1490 (3.923892, -16.14403) -> (4.11613, -16.302951)
  line L1491 (4.11613, -16.302951) -> (4.177167, -16.947413)
  line L1492 (4.018179, -17.139575) -> (4.177167, -16.947413)
  line L1493 (4.177167, -16.947413) -> (5.319402, -16.839232)
  line L1494 (5.511497, -16.998144) -> (5.319402, -16.839232)
  line L1495 (5.319402, -16.839232) -> (5.258365, -16.19477)
  circle A30 centre (4.457004, -16.595785) radius 0.1
  line L1496 (4.63234, -16.729851) -> (4.30996, -16.760383)
  line L1497 (4.30996, -16.760383) -> (4.281674, -16.46172)
  line L1498 (4.281674, -16.46172) -> (4.604054, -16.431188)
  line L1499 (4.604054, -16.431188) -> (4.63234, -16.729851)
  line L1500 (4.604068, -16.431188) -> (4.632355, -16.729852)
  line L1501 (-2.497175, -34.967272) -> (-2.49716, -34.767272)
  line L1502 (-2.49716, -34.767272) -> (-2.24716, -34.767291)
  line L1503 (-3.49716, -34.767196) -> (-3.497175, -34.967196)
  line L1504 (-3.74716, -34.767177) -> (-3.49716, -34.767196)
  line L1505 (-2.497175, -34.967272) -> (-3.497175, -34.967196)
  line L1506 (-3.74716, -34.767177) -> (-3.747015, -32.867177)
  line L1507 (-2.247015, -32.867291) -> (-2.24716, -34.767291)
  line L1508 (-3.497, -32.667196) -> (-2.497, -32.667272)
  line L1509 (-2.247015, -32.867291) -> (-2.497015, -32.867272)
  line L1510 (-2.497015, -32.867272) -> (-2.497, -32.667272)
  line L1511 (-3.497, -32.667196) -> (-3.497015, -32.867196)
  line L1512 (-3.497015, -32.867196) -> (-3.747015, -32.867177)
  line L1513 (-3.497145, -34.567196) -> (-3.497031, -33.067196)
  line L1514 (-3.497031, -33.067196) -> (-2.497031, -33.067272)
  line L1515 (-2.497031, -33.067272) -> (-2.497145, -34.567272)
  line L1516 (-2.497145, -34.567272) -> (-3.497145, -34.567196)
  line L1517 (-3.320717, -33.243536) -> (-3.320804, -34.390882)
  line L1518 (-3.497031, -33.067196) -> (-3.320717, -33.243536)
  line L1519 (-3.497145, -34.567196) -> (-3.320804, -34.390882)
  line L1520 (-3.320804, -34.390882) -> (-2.673458, -34.390931)
  line L1521 (-2.497145, -34.567272) -> (-2.673458, -34.390931)
  line L1522 (-2.673458, -34.390931) -> (-2.673371, -33.243585)
  line L1523 (-2.497031, -33.067272) -> (-2.673371, -33.243585)
  line L1524 (-2.673371, -33.243585) -> (-3.320717, -33.243536)
  circle A31 centre (-2.997108, -34.079145) radius 0.1
  line L1525 (-2.847095, -33.917245) -> (-2.84712, -34.241068)
  line L1526 (-2.84712, -34.241068) -> (-3.14712, -34.241045)
  line L1527 (-3.14712, -34.241045) -> (-3.147095, -33.917222)
  line L1528 (-3.147095, -33.917222) -> (-2.847095, -33.917245)
  line L1529 (1.153631, -24.369549) -> (0.953631, -24.369534)
  line L1530 (0.953631, -24.369534) -> (0.95365, -24.119534)
  line L1531 (0.953555, -25.369534) -> (1.153555, -25.369549)
  line L1532 (0.953536, -25.619534) -> (0.953555, -25.369534)
  line L1533 (1.153631, -24.369549) -> (1.153555, -25.369549)
  line L1534 (0.953536, -25.619534) -> (-0.946464, -25.61939)
  line L1535 (-0.94635, -24.11939) -> (0.95365, -24.119534)
  line L1536 (-1.146445, -25.369375) -> (-1.146369, -24.369375)
  line L1537 (-0.94635, -24.11939) -> (-0.946369, -24.36939)
  line L1538 (-0.946369, -24.36939) -> (-1.146369, -24.369375)
  line L1539 (-1.146445, -25.369375) -> (-0.946445, -25.36939)
  line L1540 (-0.946445, -25.36939) -> (-0.946464, -25.61939)
  line L1541 (0.753555, -25.369519) -> (-0.746445, -25.369405)
  line L1542 (-0.746445, -25.369405) -> (-0.746369, -24.369405)
  line L1543 (-0.746369, -24.369405) -> (0.753631, -24.369519)
  line L1544 (0.753631, -24.369519) -> (0.753555, -25.369519)
  line L1545 (-0.570105, -25.193091) -> (0.577241, -25.193179)
  line L1546 (-0.746445, -25.369405) -> (-0.570105, -25.193091)
  line L1547 (0.753555, -25.369519) -> (0.577241, -25.193179)
  line L1548 (0.577241, -25.193179) -> (0.57729, -24.545833)
  line L1549 (0.753631, -24.369519) -> (0.57729, -24.545833)
  line L1550 (0.57729, -24.545833) -> (-0.570056, -24.545745)
  line L1551 (-0.746369, -24.369405) -> (-0.570056, -24.545745)
  line L1552 (-0.570056, -24.545745) -> (-0.570105, -25.193091)
  circle A32 centre (0.265504, -24.869482) radius 0.1
  line L1553 (0.103604, -24.71947) -> (0.427427, -24.719494)
  line L1554 (0.427427, -24.719494) -> (0.427404, -25.019494)
  line L1555 (0.427404, -25.019494) -> (0.103581, -25.01947)
  line L1556 (0.103581, -25.01947) -> (0.103604, -24.71947)
  line L1557 (3.502825, -34.967728) -> (3.50284, -34.767728)
  line L1558 (3.50284, -34.767728) -> (3.75284, -34.767747)
  line L1559 (2.50284, -34.767652) -> (2.502825, -34.967652)
  line L1560 (2.25284, -34.767633) -> (2.50284, -34.767652)
  line L1561 (3.502825, -34.967728) -> (2.502825, -34.967652)
  line L1562 (2.25284, -34.767633) -> (2.252985, -32.867633)
  line L1563 (3.752985, -32.867747) -> (3.75284, -34.767747)
  line L1564 (2.503, -32.667652) -> (3.503, -32.667728)
  line L1565 (3.752985, -32.867747) -> (3.502985, -32.867728)
  line L1566 (3.502985, -32.867728) -> (3.503, -32.667728)
  line L1567 (2.503, -32.667652) -> (2.502985, -32.867652)
  line L1568 (2.502985, -32.867652) -> (2.252985, -32.867633)
  line L1569 (2.502855, -34.567652) -> (2.502969, -33.067652)
  line L1570 (2.502969, -33.067652) -> (3.502969, -33.067728)
  line L1571 (3.502969, -33.067728) -> (3.502855, -34.567728)
  line L1572 (3.502855, -34.567728) -> (2.502855, -34.567652)
  line L1573 (2.679283, -33.243993) -> (2.679196, -34.391339)
  line L1574 (2.502969, -33.067652) -> (2.679283, -33.243993)
  line L1575 (2.502855, -34.567652) -> (2.679196, -34.391339)
  line L1576 (2.679196, -34.391339) -> (3.326542, -34.391388)
  line L1577 (3.502855, -34.567728) -> (3.326542, -34.391388)
  line L1578 (3.326542, -34.391388) -> (3.326629, -33.244042)
  line L1579 (3.502969, -33.067728) -> (3.326629, -33.244042)
  line L1580 (3.326629, -33.244042) -> (2.679283, -33.243993)
  circle A33 centre (3.002892, -34.079602) radius 0.1
  line L1581 (3.152905, -33.917702) -> (3.15288, -34.241524)
  line L1582 (3.15288, -34.241524) -> (2.85288, -34.241502)
  line L1583 (2.85288, -34.241502) -> (2.852905, -33.917679)
  line L1584 (2.852905, -33.917679) -> (3.152905, -33.917702)
  line L1585 (3.439956, -6.946341) -> (3.439941, -7.145255)
  line L1586 (3.439941, -7.145255) -> (3.689941, -7.145274)
  line L1587 (2.439941, -7.145179) -> (2.439956, -6.946265)
  line L1588 (2.189941, -7.14516) -> (2.439941, -7.145179)
  line L1589 (3.439956, -6.946341) -> (2.439956, -6.946265)
  line L1590 (2.189941, -7.14516) -> (2.189807, -8.903105)
  line L1591 (3.689807, -8.903219) -> (3.689941, -7.145274)
  line L1592 (2.439926, -7.344093) -> (2.439822, -8.704473)
  line L1593 (3.439926, -7.344169) -> (2.439926, -7.344093)
  line L1594 (3.439822, -8.704549) -> (3.439926, -7.344169)
  line L1595 (2.439926, -7.344093) -> (2.599867, -7.59761)
  line L1596 (3.439926, -7.344169) -> (3.279945, -7.597661)
  ellipse E659 centre (2.939883, -7.907623) end of major axis (2.839883, -7.907615) minor radius 0.099457
  ellipse E660 centre (2.939882, -7.912827) end of major axis (2.839882, -7.912819) minor radius 0.099457 (2.839882, -7.912819) -> (3.039882, -7.912834) ccw
  line L1597 (3.039883, -7.907631) -> (3.039882, -7.912834)
  line L1598 (2.839883, -7.907615) -> (2.839882, -7.912819)
  line L1599 (3.08987, -8.07387) -> (3.089895, -7.751806)
  line L1600 (3.089869, -8.084417) -> (3.08987, -8.07387)
  line L1601 (3.089895, -7.751806) -> (2.789895, -7.751783)
  line L1602 (2.789895, -7.751783) -> (2.78987, -8.073847)
  line L1603 (2.789869, -8.084394) -> (2.78987, -8.073847)
  line L1604 (2.78987, -8.073847) -> (3.08987, -8.07387)
  line L1605 (7.786503, -8.278524) -> (7.765717, -8.079707)
  line L1606 (7.765717, -8.079707) -> (7.765489, -8.079631)
  line L1607 (7.765489, -8.079631) -> (7.786286, -8.278547)